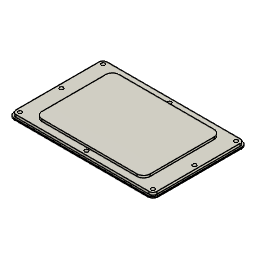
Display Mount - Blank (Autodesk Fusion 360 design; units mm, degrees)
Autodesk Fusion 360 part; units mm, degrees
note: some values were not read from the file. Set by a fixed rule: which sketch regions a step uses.
sketch "Sketch1" plane through (0, 0, 0) normal (0, 0, 1) x (1, 0, 0)
  circle A0 centre (-81.65, 51) radius 2.3
  circle A1 centre (81.65, 51) radius 2.3
  circle A2 centre (-81.65, -51) radius 2.3
  circle A3 centre (81.65, -51) radius 2.3
  line L0 (-81.65, 51) -> (81.65, 51) construction
  line L1 (81.65, 51) -> (81.65, -51) construction
  line L2 (81.65, -51) -> (-81.65, -51) construction
  line L3 (-81.65, -51) -> (-81.65, 51) construction
  circle A4 centre (-81.65, 0) radius 2.3
  circle A5 centre (0, 51) radius 2.3
  circle A6 centre (81.65, 0) radius 2.3
  circle A7 centre (0, -51) radius 2.3
  line L4 (0, 87.0412) -> (0, 82.962)
  line L5 (0, 82.962) -> (0, -82.962) construction
  line L6 (-123.3001, 0) -> (123.3001, 0) construction
  circle A8 centre (81.65, -51) radius 4.9
  circle A9 centre (-81.65, -51) radius 4.9
  circle A10 centre (-81.65, 51) radius 4.9
  circle A11 centre (81.65, 51) radius 4.9
  line L7 (-81.65, 55.9) -> (81.65, 55.9)
  line L8 (86.55, 51) -> (86.55, -51)
  line L9 (-81.65, -55.9) -> (-65.5347, -55.9)
  line L10 (-65.5347, -55.9) -> (81.65, -55.9)
  line L11 (-86.55, 51) -> (-86.55, -51)
  point P0 (0, 51)
  point P1 (81.65, 0)
  point P2 (0, -51)
  point P3 (-81.65, 0)
  dimension "d23" = 4.6
  dimension "d24" = 4.6
  dimension "d25" = 4.6
  dimension "d26" = 4.6
  dimension "d92" = 4.6
  dimension "d93" = 4.6
  dimension "d94" = 4.6
  dimension "d95" = 4.6
  dimension "d178" = 163.3
  dimension "d179" = 102
  dimension "d180" = 9.8
  dimension "d181" = 9.8
  dimension "d182" = 9.8
  dimension "d183" = 9.8
  constraint coincident A0.centre L0.start
  constraint coincident A3.centre L1.end
  constraint coincident A2.centre L2.end
  constraint midpoint L0 P0
  constraint midpoint L1 P1
  constraint midpoint L2 P2
  constraint midpoint L3 P3
  constraint coincident P3 A4.centre
  constraint coincident P0 A5.centre
  constraint coincident P1 A6.centre
  constraint coincident P2 A7.centre
  constraint midpoint origin L6
  constraint midpoint origin L5
  constraint symmetric A0.centre A1.centre L5
  constraint vertical A0.centre P3
  constraint symmetric A0.centre A2.centre L6
  constraint coincident P1 L6
  constraint parallel L0 L2
  constraint parallel L1 L3
  constraint coincident P0 L5
  constraint concentric A3 A8
  constraint concentric A2 A9
  constraint concentric A0 A10
  constraint concentric A1 A11
  constraint coincident A10 L7.start
  constraint coincident A11 L7.end
  constraint parallel L0 L7
  constraint tangent A11 L7
  constraint coincident A11 L8.start
  constraint coincident A8 L8.end
  constraint vertical L8
  constraint tangent A8 L8
  constraint coincident A9 L9.start
  constraint tangent A9 L9
  constraint perpendicular L5 L9
  constraint coincident A8 L10.end
  constraint tangent A8 L10
  constraint perpendicular L5 L10
  constraint coincident A10 L11.start
  constraint coincident A9 L11.end
  constraint tangent A9 L11
  constraint tangent A10 L11
  measures "d23" diameter of A0
  measures "d24" diameter of A1
  measures "d25" diameter of A2
  measures "d26" diameter of A3
  measures "d92" diameter of A4
  measures "d93" diameter of A7
  measures "d94" diameter of A6
  measures "d95" diameter of A5
  measures "d178" distance of A0.centre A1.centre
  measures "d179" distance of A0.centre A2.centre
  measures "d180" diameter of A8
  measures "d181" diameter of A9
  measures "d182" diameter of A10
  measures "d183" diameter of A11
extrude "Extrude1" add sketch "Sketch1" along normal blind 3
sketch "Sketch6" plane through (0, 0, 3) normal (0, 0, 1) x (-1, 0, 0)
  circle A0 centre (-81.65, 51) radius 2.3
  circle A1 centre (-81.65, -51) radius 2.3
  circle A2 centre (81.65, -51) radius 2.3
  circle A3 centre (81.65, 51) radius 2.3
  line L0 (0, -100) -> (0, 100) construction
  line L1 (148.8555, 0) -> (144.6445, 0)
  line L2 (144.6445, 0) -> (-144.6445, 0) construction
  line L3 (66.4, -47.3125) -> (-66.4, -47.3125)
  line L4 (-66.4, -47.3125) -> (-66.4, 47.3125)
  line L5 (-66.4, 47.3125) -> (66.4, 47.3125)
  line L6 (66.4, 47.3125) -> (66.4, -47.3125)
  circle A4 centre (0, 51) radius 2.3
  circle A5 centre (81.65, 0) radius 2.3
  circle A6 centre (0, -51) radius 2.3
  circle A7 centre (-81.65, 0) radius 2.3
  arc A8 (-81.65, 55.9) -> (-86.55, 51) centre (-81.65, 51) ccw
  arc A9 (-86.55, -51) -> (-81.65, -55.9) centre (-81.65, -51) ccw
  arc A10 (81.65, -55.9) -> (86.55, -51) centre (81.65, -51) ccw
  arc A11 (86.55, 51) -> (81.65, 55.9) centre (81.65, 51) ccw
  line L7 (-81.65, -55.9) -> (81.65, -55.9)
  line L8 (86.55, -51) -> (86.55, 51)
  line L9 (81.65, 55.9) -> (-81.65, 55.9)
  line L10 (-86.55, 51) -> (-86.55, -51)
  constraint vertical L0
  constraint horizontal L1
  constraint midpoint origin L2
  constraint midpoint origin L0
  constraint horizontal L3
  constraint vertical L4
  constraint horizontal L5
  constraint vertical L6
  constraint symmetric L0 L4 L6
  constraint symmetric L2 L3 L5
extrude "Extrude7" add sketch "Sketch6" along normal blind 2.6 contours L3 L4 L5 L6
fillet "Fillet2" radius 8 4 edges at (-66.4, -47.3125, 4.3) (66.4, -47.3125, 4.3) (66.4, 47.3125, 4.3) (-66.4, 47.3125, 4.3)
sketch "Sketch8" plane through (0, 0, 0) normal (0, 0, -1) x (1, 0, 0)
  circle A0 centre (81.65, 51) radius 2.3
  circle A1 centre (0, 51) radius 2.3
  circle A2 centre (-81.65, 0) radius 2.3
  circle A3 centre (-81.65, 51) radius 2.3
  circle A4 centre (81.65, -51) radius 2.3
  circle A5 centre (0, -51) radius 2.3
  circle A6 centre (-81.65, -51) radius 2.3
  circle A7 centre (81.65, 0) radius 2.3
  line L0 (81.65, 57.9) -> (-81.65, 57.9)
  line L1 (-88.55, 51) -> (-88.55, -51)
  line L2 (-81.65, -57.9) -> (81.65, -57.9)
  line L3 (88.55, -51) -> (88.55, 51)
  arc A8 (86.55, 51) -> (81.65, 55.9) centre (81.65, 51) ccw
  arc A9 (-81.65, 55.9) -> (-86.55, 51) centre (-81.65, 51) ccw
  arc A10 (-86.55, -51) -> (-81.65, -55.9) centre (-81.65, -51) ccw
  arc A11 (81.65, -55.9) -> (86.55, -51) centre (81.65, -51) ccw
  line L4 (86.55, -51) -> (86.55, 51)
  line L5 (81.65, 55.9) -> (-81.65, 55.9)
  line L6 (-86.55, 51) -> (-86.55, -51)
  line L7 (-81.65, -55.9) -> (81.65, -55.9)
  circle A12 centre (81.65, 51) radius 6.9
  circle A13 centre (-81.65, 51) radius 6.9
  circle A14 centre (-81.65, -51) radius 6.9
  circle A15 centre (81.65, -51) radius 6.9
  dimension "d184" = 2
  dimension "d185" = 2
  dimension "d186" = 2
  dimension "d187" = 2
  constraint concentric A0 A12
  constraint tangent L3 A12
  constraint tangent L0 A13
  constraint tangent L1 A13
  constraint coincident A3.centre A9.centre
  constraint tangent L1 A14
  constraint tangent L2 A14
  constraint coincident A6.centre A10.centre
  constraint tangent L2 A15
  constraint tangent L3 A15
  constraint coincident A4.centre A11.centre
  constraint coincident L0.end A13
  constraint coincident L0.start A12
  constraint coincident L2.end A15
  constraint coincident L2.start A14
  constraint coincident L1.start A13
  constraint coincident L1.end A14
  constraint coincident L3.start A15
  constraint coincident L3.end A12
  measures "d184" distance of L1 L6
  measures "d185" distance of L0 L5
  measures "d186" distance of L3 L4
  measures "d187" distance of L2 L7
extrude "Extrude15" add sketch "Sketch8" along normal blind 2.4
fillet "Fillet5" radius 1 8 edges at (88.55, 0, -2.4) (86.529, -55.879, -2.4) (0, -57.9, -2.4) (-86.529, -55.879, -2.4) (-88.55, 0, -2.4) (-86.529, 55.879, -2.4) (0, 57.9, -2.4) (86.529, 55.879, -2.4)
equation "d24 = d23"
equation "d25 = d23"
equation "d26 = d23"
equation "d92 = d23"
equation "d93 = d23"
equation "d94 = d23"
equation "d95 = d23"
equation "d178 = 173.2 mm - 9.9 mm"
equation "d180 = d181"
equation "d182 = d181"
equation "d183 = d181"
